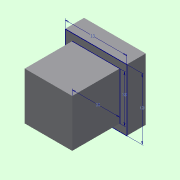
# Autodesk Inventor part: Cuvette_cover
Saved by Autodesk Inventor 2015 (Build 190159000, 159)
## iProperties
Created: 2015-05-26
Part Number: Cuvette_cover
Material: Generic
Document SubType Name: Modeling
Designer: Openlab
Density: 1 g/cm^3
Appearance: Default
Author: Openlab
Autodesk Inventor part; units mm, degrees
ref_plane "YZ Plane" through (0, 0, 0) normal (1, 0, 0) x (0, 1, 0)
ref_plane "XZ Plane" through (0, 0, 0) normal (0, 1, 0) x (-1, 0, 0)
ref_plane "XY Plane" through (0, 0, 0) normal (0, 0, 1) x (1, 0, 0)
sketch "Sketch1" plane through (0, 0, 0) normal (0, 1, 0) x (-1, 0, 0)
  line L0 (0, 0) -> (13, 0)
  line L1 (13, 0) -> (13, -13)
  line L2 (13, -13) -> (0, -13)
  line L3 (0, -13) -> (0, 0)
  line L4 (11.5, -1.5) -> (1.5, -1.5)
  line L5 (1.5, -1.5) -> (1.5, -11.5)
  line L6 (1.5, -11.5) -> (11.5, -11.5)
  line L7 (11.5, -11.5) -> (11.5, -1.5)
  line L8 (6.5, -3.7136) -> (6.5, -8.8552) construction
  line L9 (8.9776, -6.5) -> (3.1629, -6.5) construction
  dimension "d10" = 13
  dimension "d11" = 13
  dimension "d12" = 10
  dimension "d13" = 10
  constraints: 20 end point, 4 parallel, 3 horizontal, 2 perpendicular, 4 other
  measures "d10" distance of L0.start L0.end
  measures "d11" distance of L2.end L0.start
  measures "d12" distance of L5.end L6.end
  measures "d13" distance of L4.end L5.end
extrude "Extrusion3" add sketch "Sketch1" along normal blind 4 contours L0 L1 L2 L3 | L7 L6 L5 L4
extrude "Extrusion5" add sketch "Sketch1" against normal blind 10 contours L7 L6 L5 L4
body "Solid2"
